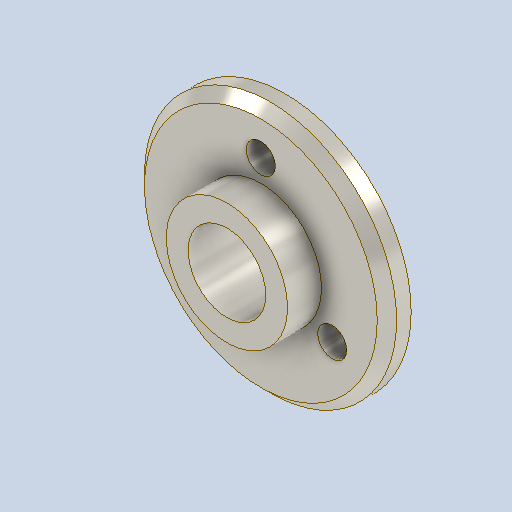
# Autodesk Inventor part: EndBush
Saved by Autodesk Inventor 2023.2 (Build 272271030, 271C)
## iProperties
Created: 2023-03-30
Part Number: EndBush
Material: Titanium
Document SubType Name: Modeling
Designer: Luis Valente
Density: 4.51 g/cm^3
Appearance: Titanium
Author: Luis Valente
Autodesk Inventor part; units mm, degrees
ref_plane "YZ Plane" through (0, 0, 0) normal (1, 0, 0) x (0, 1, 0)
sketch "Sketch1" plane through (0, 0, 0) normal (0, 0, 1) x (1, 0, 0)
  circle A0 centre (0, 0) radius 26
  dimension "d0" = 52
  constraints: 1 centre point, 1 coincident
  measures "d0" diameter of A0
extrude "Extrusion1" add sketch "Sketch1" along normal blind 5
chamfer "Chamfer2" distance 2 angle 45 1 edges at (-26, 0, 5)
ref_plane "Work Plane3" through (0, 0, 5) normal (0, 0, 1) x (1, 0, 0)
sketch "Sketch3" plane through (0, 0, 5) normal (0, 0, 1) x (1, 0, 0)
  circle A0 centre (0, 0) radius 12.5
  dimension "d6" = 25
  constraints: 1 centre point, 1 coincident
  measures "d6" diameter of A0
extrude "Extrusion2" add sketch "Sketch3" along normal blind 7
ref_plane "Work Plane4" through (0, 0, 12) normal (0, 0, 1) x (1, 0, 0)
sketch "Sketch4" plane through (0, 0, 12) normal (0, 0, 1) x (1, 0, 0)
  circle A0 centre (0, 0) radius 8
  dimension "d9" = 16
  constraints: 1 centre point, 1 coincident
  measures "d9" diameter of A0
extrude "Extrusion3" cut sketch "Sketch4" against normal blind 12
sketch "Sketch2" plane through (0, 0, 0) normal (0, 0, -1) x (-1, 0, 0)
  line L0 (0, 0) -> (-23.1702, 23.1702)
  line L1 (0, 0) -> (32.7676, 0) construction
  line L2 (-23.1702, 23.1702) -> (18.3848, -18.3848)
  circle A0 centre (0, 0) radius 26 projected
  line L3 (0, 0) -> (-21.488, -21.488)
  line L4 (0, 0) -> (30.3887, 0) construction
  line L5 (-21.488, -21.488) -> (18.3848, 18.3848)
  circle A1 centre (0, 0) radius 8 projected
  line L6 (0, 8) -> (0, 17)
  circle A2 centre (0, 17) radius 3
  line L7 (0, -26) -> (0, 26)
  circle A3 centre (-14.7224, -8.5) radius 3
  circle A4 centre (14.7224, -8.5) radius 3
  dimension "d4" = 135
  dimension "d5" = 135
  dimension "d19" = 9
  dimension "d20" = 6
  dimension "d23" = 360
  constraints: 16 end point, 4 point on circle, 3 centre point, 2 equal length, 2 horizontal, 2 point on line, 2 vertical, 1 coincident, 1 vertical alignment, 8 other
  measures "d4" angle of L1 L0
  measures "d5" angle of L3 L4
  measures "d19" distance of L6.start L6.end
  measures "d20" diameter of A2
extrude "Extrusion4" cut sketch "Sketch2" against normal blind 12 contours A2 L7 L6 | L6 L7 A2 | A3 | A4
body "Solid1"
